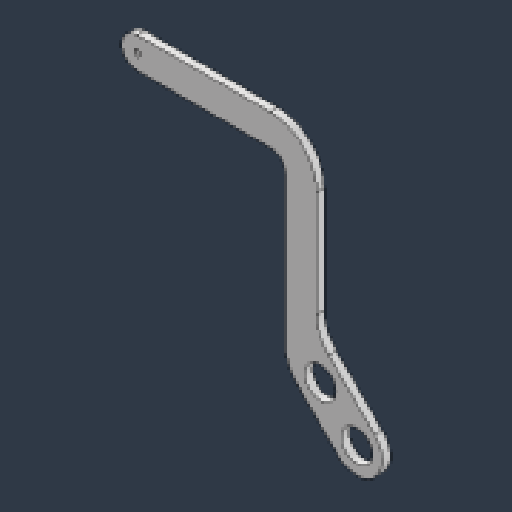
# Autodesk Inventor part: ARM,KICKER
Saved by Autodesk Inventor 2026 (Build 300175050, 175E)
## iProperties
Created: 2026-04-12
Part Number: ARM,KICKER
Material: Generic
Document SubType Name: Sheet Metal
Designer: Jthib
Mass: 25.3 g
Surface Area: 139.945 cm^2
Volume: 25.3 cm^3
Density: 1 g/cm^3
Appearance: Default
Sheet Metal Rule: Default
Author: Jthib
Autodesk Inventor part; units mm, degrees
ref_plane "YZ Plane" through (0, 0, 0) normal (1, 0, 0) x (0, 1, 0)
ref_plane "XZ Plane" through (0, 0, 0) normal (0, 1, 0) x (-1, 0, 0)
ref_plane "XY Plane" through (0, 0, 0) normal (0, 0, 1) x (1, 0, 0)
sketch "Sketch1" plane through (0, 0, 0) normal (0, 0, 1) x (1, 0, 0)
  circle A0 centre (0, 0) radius 9.525
  line L0 (0, 9.525) -> (81.915, 9.525)
  arc A1 (110.49, -19.05) -> (81.915, 9.525) centre (81.915, -19.05) ccw
  line L1 (110.49, -19.05) -> (110.49, -94.7987)
  line L2 (110.49, -94.7987) -> (146.411, -130.7197)
  arc A2 (123.9604, -153.1704) -> (146.411, -130.7197) centre (135.1857, -141.9451) ccw
  line L3 (123.9604, -153.1704) -> (91.44, -120.65)
  line L4 (91.44, -120.65) -> (91.44, -19.05)
  arc A3 (91.44, -19.05) -> (81.915, -9.525) centre (81.915, -19.05) ccw
  line L5 (81.915, -9.525) -> (0, -9.525)
  circle A4 centre (135.1857, -141.9451) radius 9.525
  circle A5 centre (112.7351, -119.4944) radius 9.525
  line L6 (135.1857, -141.9451) -> (112.7351, -119.4944) construction
  dimension "d0" = 19.05
  dimension "d1" = 9.525
  dimension "d4" = 91.44
  dimension "d5" = 101.6
  dimension "d6" = 31.75
  dimension "d7" = 50.8
  dimension "d8" = 19.05
  dimension "d9" = 19.05
  dimension "d10" = 31.75
  dimension "d11" = 135
  constraints: 14 end point, 8 point on circle, 8 tangent, 6 centre point, 3 parallel, 2 coincident, 2 perpendicular, 1 concentric, 1 horizontal
  measures "d0" diameter of A0
  measures "d1" radius of A3
  measures "d4" distance from line of L4 point (0, 0)
  measures "d5" distance of L3.end L4.end
  measures "d6" distance between parallel lines of L2 L3
  measures "d7" distance of L1.end L2.end
  measures "d8" diameter of A4
  measures "d9" diameter of A5
  measures "d10" distance of L6.start L6.end
  measures "d11" angle of L1 L2
extrude "Extrusion1" add sketch "Sketch1" along normal blind 4.7625
sketch "Sketch2" plane through (0, 0, 4.7625) normal (0, 0, 1) x (1, 0, 0)
  arc A0 (0, 9.525) -> (0, -9.525) centre (0, 0) ccw construction
  constraints: 1 coincident
hole "Hole1" at (0, 0, 4.7625) direction (0, 0, -1) diameter 3.9624 end through all thread size "10-32 UNF" class "2B" standard "ANSI Unified Screw Threads"
fillet "Fillet1" radius 25.4 2 edges at (110.49, -94.7987, 2.3813) (91.44, -120.65, 2.3813)
equation "\"BendRadius\" = Thickness"
equation "\"BendReliefWidth\" = Thickness"
equation "\"BendReliefDepth\" = 0.5 * Thickness"
equation "\"CornerReliefSize\" = 4 * Thickness"
equation "\"MinimumRemnant\" = 2 * Thickness"
equation "\"TransitionRadius\" = BendRadius"
equation "\"JacobiRadiusSize\" = BendRadius"
equation "\"GapSize\" = Thickness"
equation "\"Thickness\" = 3.048"
body "Solid1"
